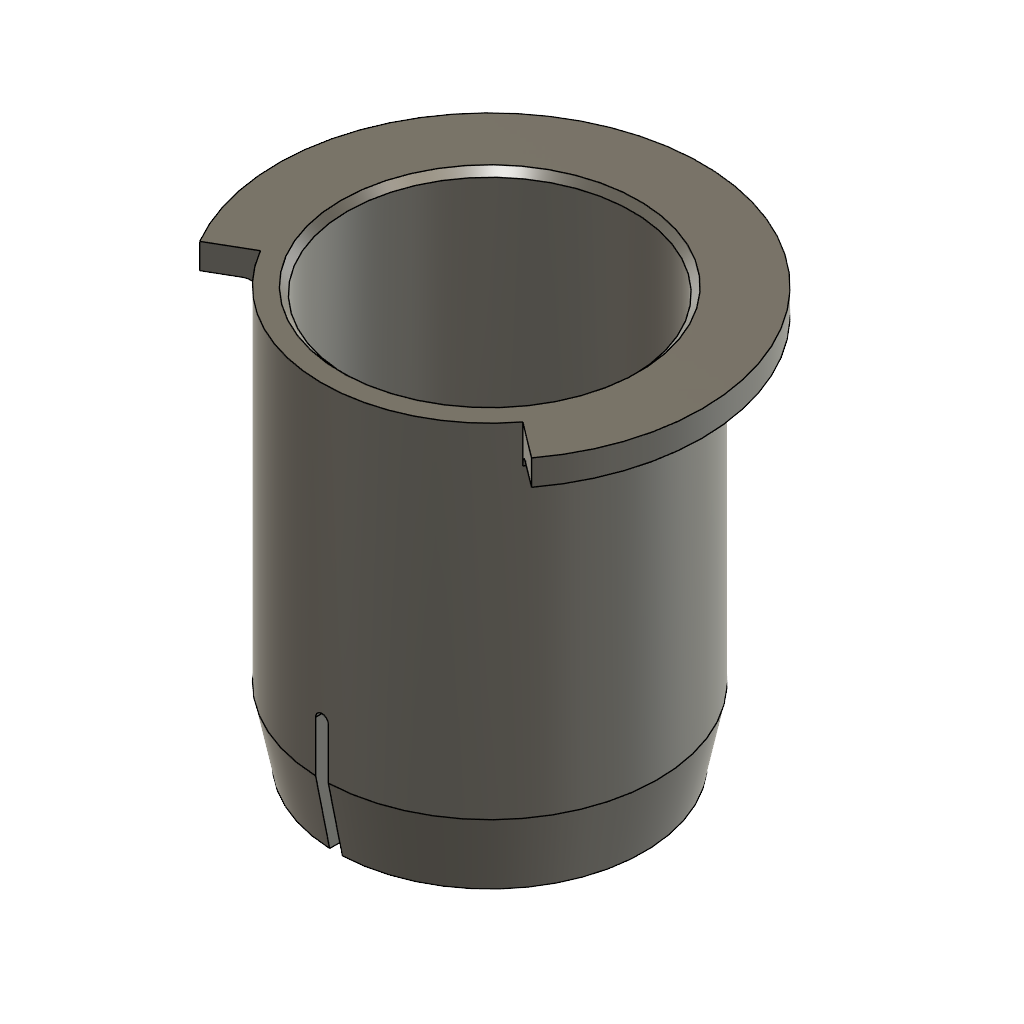
LEE MEASURE VALVE (Autodesk Fusion 360 design; units mm, degrees)
part number: 2026-09-15-09-17-11-328
Autodesk Fusion 360 part; units mm, degrees
sketch "Sketch1" plane through (0, 0, 0) normal (0, 1, 0) x (1, 0, 0)
  circle A0 centre (0, 0) radius 11.2
  circle A1 centre (0, 0) radius 13.2
  line L0 (13.2, 0) -> (7.875, 9.2232)
  line L1 (7.875, 9.2232) -> (-2.775, 9.2232)
  line L2 (-2.775, 9.2232) -> (-8.1, 0)
  line L3 (-8.1, 0) -> (-2.775, -9.2232)
  line L4 (-2.775, -9.2232) -> (7.875, -9.2232)
  line L5 (7.875, -9.2232) -> (13.2, 0)
  line L6 (10.85, 0) -> (6.7, 7.188)
  line L7 (6.7, 7.188) -> (-1.6, 7.188)
  line L8 (-1.6, 7.188) -> (-5.75, 0)
  line L9 (-5.75, 0) -> (-1.6, -7.188)
  line L10 (-1.6, -7.188) -> (6.7, -7.188)
  line L11 (6.7, -7.188) -> (10.85, 0)
  circle A2 centre (5.9425, 0) radius 4.25
  circle A3 centre (0, 0) radius 16.7
  line L12 (0, 0) -> (13.3372, -10.0503)
  line L13 (0, 0) -> (16.7, 0) construction
  line L14 (0, 0) -> (-14.4626, -8.35)
  point P0 (11.2, 0)
  point P1 (2.55, 0)
  point P2 (13.2, 0)
  point P3 (2.55, 0)
  dimension "d1" = 22.4
  dimension "d2" = 26.4
  dimension "d3" = 10.65
  dimension "d4" = 8.3
  dimension "d5" = 8.5
  dimension "d12" = 33.4
  dimension "d17" = 37
  dimension "d18" = 67
  constraint coincident A0.centre A1.centre
  constraint concentric A0 A1
  constraint coincident A0 P0
  constraint coincident A1 P2
  constraint coincident P3 P1
  constraint horizontal L13
  constraint coincident A3 L12.end
  constraint coincident A3 L14.end
  measures "d1" diameter of A0
  measures "d2" diameter of A1
  measures "d3" distance of P2 P3
  measures "d4" distance of L6.start P3
  measures "d5" diameter of A2
  measures "d12" diameter of A3
  measures "d17" angle of L12 L13
  measures "d18" angle of L12 L14
extrude "Extrude1" add sketch "Sketch1" against normal blind 2 contours A0 L1 L2 L3 L6 L7 L8 L9 L11 L12 L14 | A0 L0 L1 L5 L12 | A0 L1 L2 L3 L14 | A0 A1 L0 L1 L14 | A0 L4 L5 L12 | A0 L3 L4 L9 L10 L11 L12 L14 | A0 L3 L4 L14 | A0 A1 L4 L5 L12 L14 | L11 A2 L12 | L9 L10 L11 A2 L12 L14 | A1 L5 L12 | L6 L11 A2 | L6 L7 L8 L9 A2 L12 L14
extrude "Extrude2" add sketch "Sketch1" along normal blind 19.5 contours A0 L0 L1 L5 L12 | A0 A1 L0 L1 L14 | A0 L4 L5 L12 | A0 A1 L4 L5 L12 L14 | A1 L5 L12
extrude "Extrude4" add sketch "Sketch1" along normal blind 19.5 and the other way blind -17.5 contours A1 A3 L12 L14 picked at (-14.8791, -4.3251)
sketch "Sketch2" plane through (0, 0, 0) normal (0, 1, 0) x (1, 0, 0)
  circle A0 centre (0, 0) radius 10.05
  circle A1 centre (0, 0) radius 13.2
  line L0 (0, 10.05) -> (-8.7036, -5.025)
  line L1 (-8.7036, -5.025) -> (8.7036, -5.025)
  line L2 (8.7036, -5.025) -> (0, 10.05)
  circle A2 centre (0, 10.05) radius 0.5
  circle A3 centre (-8.7036, -5.025) radius 0.5
  circle A4 centre (8.7036, -5.025) radius 0.5
  dimension "d19" = 20.1
  dimension "d20" = 26.4
  dimension "d37" = 10.05
  dimension "d38" = 1
  dimension "d39" = 1
  dimension "d40" = 1
  constraint coincident A0.centre A1.centre
  constraint concentric A0 A1
  constraint coincident L0.start L2.end
  constraint coincident L0.end L1.start
  constraint coincident L1.end L2.start
  measures "d19" diameter of A0
  measures "d20" diameter of A1
  measures "d37" distance of L0.start A0.centre
  measures "d38" diameter of A2
  measures "d39" diameter of A3
  measures "d40" diameter of A4
extrude "Extrude5" add sketch "Sketch2" against normal blind 13 contours A0 A2 | A0 A4 | A0 A3 | A1
sketch "Sketch3" plane through (0, 0, 0) normal (0, 0, 1) x (1, 0, 0)
  line L0 (0, -2) -> (0, -13)
  line L1 (0.5, -2) -> (-0.5, -2)
  line L2 (-0.5, -2) -> (-0.5, -13)
  line L3 (-0.5, -13) -> (0.5, -13)
  line L4 (0.5, -13) -> (0.5, -2)
  line L5 (0.5, -2) -> (-0.5, -13) construction
  line L6 (-0.5, -2) -> (0.5, -13) construction
  line L7 (0.5, -3) -> (-0.5, -3)
  line L8 (-0.5, -3) -> (-0.5, -12)
  line L9 (-0.5, -12) -> (0.5, -12)
  line L10 (0.5, -12) -> (0.5, -3)
  line L11 (0.5, -3) -> (-0.5, -12) construction
  line L12 (-0.5, -3) -> (0.5, -12) construction
  point P0 (0, -7.5)
  point P1 (0, -7.5)
  dimension "d24" = 1
  dimension "d25" = 11
  dimension "d26" = 1
  dimension "d27" = 9
  constraint vertical L0
  constraint horizontal L1
  constraint perpendicular L1 L2
  constraint parallel L1 L3
  constraint parallel L2 L4
  constraint coincident L5 P1
  constraint coincident L6 P1
  constraint midpoint L0 P1
  constraint horizontal L7
  constraint perpendicular L7 L8
  constraint parallel L7 L9
  constraint parallel L8 L10
  constraint coincident L11 P1
  constraint coincident L12 P1
  constraint coincident P1 P0
  measures "d24" distance of L2.end L3.end
  measures "d25" distance of L1.end L2.end
  measures "d26" distance of L8.end L9.end
  measures "d27" distance of L7.end L8.end
extrude "Extrude6" cut sketch "Sketch3" along normal blind 13.2 contours L0 L4 L7 L9 L10 | L0 L2 L7 L8 L9 | L0 L3 L4 L9 | L0 L2 L3 L9
extrude "Extrude7" add sketch "Sketch2" against normal blind 12 contours A0 L2 A2 | A0 L2 A4 | A0 L0 A2 | L0 L2 A2 | A0 L1 A4 | L1 L2 A4 | A0 L0 A3 | L0 L1 A3 | A0 L1 A3
chamfer "Chamfer1" distance 1 angle 45 1 edges at (-9.3699, -13, 3.6342)
fillet "Fillet1" radius 0.5 2 edges at (-0.5, -3, 11.614) (0.5, -3, 11.614)
chamfer "Chamfer2" distance 0.5 angle 45 1 edges at (-10.4421, 19.5, -4.0501)
fillet "Fillet2" radius 1 2 edges at (0.8058, 17.5, -13.1754) (-10.4421, 0, 4.0501)
chamfer "Chamfer3" distance 1.1 distance2 5.5 1 edges at (0, -13, -13.2) measured on face at (12.4193, -13, -0.9948)
chamfer "Chamfer4" distance 0.5 distance2 1 3 edges at (-8.2705, -12, 4.775) (0, -12, -9.55) (8.2705, -12, 4.775) measured on face at (-8.5649, -12, 4.9308) measured on face at (0.0123, -12, -9.8829) measured on face at (8.5527, -12, 4.952)
extrude "Extrude3" [suppressed]
equation "d2 = d1 + 4 mm"
equation "d3 = ( 21.3 / 2 ) * 1 mm"
equation "d4 = ( 16.6 / 2 ) * 1 mm"
equation "d10 = -2.00 mm - 17.5 mm"
equation "d12 = d2 + 7 mm"
equation "d15 = -19.50 mm + 2 mm"
equation "d20 = d2"
equation "d21 = -2.00 mm - 11 mm"
equation "d27 = 11 mm - 2 mm"
equation "d28 = d2 / 2"
equation "d37 = d19 / 2"
equation "d39 = d38"
equation "d40 = d38"
